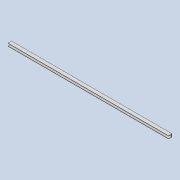
# Autodesk Inventor part: Decupare Heated Bed
Saved by Autodesk Inventor 2020 (Build 240168000, 168)
## iProperties
Created: 2021-01-16
Part Number: Decupare Heated Bed
Material: Generic
Document SubType Name: Modeling
Designer: Iulian Bors
Density: 1 g/cm^3
Appearance: Default
Author: Iulian Bors
Autodesk Inventor part; units mm, degrees
ref_plane "YZ Plane" through (0, 0, 0) normal (1, 0, 0) x (0, 1, 0)
ref_plane "XZ Plane" through (0, 0, 0) normal (0, 1, 0) x (-1, 0, 0)
ref_plane "XY Plane" through (0, 0, 0) normal (0, 0, 1) x (1, 0, 0)
sketch "Sketch1" plane through (0, 0, 0) normal (0, 0, 1) x (1, 0, 0)
  line L0 (-115, 2) -> (115, 2)
  line L1 (115, 2) -> (115, -2)
  line L2 (115, -2) -> (-115, -2)
  line L3 (-115, -2) -> (-115, 2)
  point P0 (0, 0)
  point P1 (-115, 0)
  point P2 (0, 2)
  dimension "d0" = 230
  dimension "d1" = 4
  constraints: 8 end point, 2 midpoint, 2 parallel, 1 horizontal, 1 horizontal alignment, 1 perpendicular, 1 vertical alignment
  measures "d0" distance of L0.start L0.end
  measures "d1" distance of L2.end L0.start
extrude "Extrusion1" add sketch "Sketch1" along normal blind 5
sketch "Sketch2" plane through (0, 0, 5) normal (0, 0, 1) x (1, 0, 0)
  line L0 (-118.277, 1.6) -> (118.277, 1.6)
  line L1 (118.277, 1.6) -> (118.277, -1.6)
  line L2 (118.277, -1.6) -> (-118.277, -1.6)
  line L3 (-118.277, -1.6) -> (-118.277, 1.6)
  point P0 (0, 0)
  point P1 (0, 1.6)
  point P2 (-118.277, 0)
  dimension "d4" = 3.2
  constraints: 8 end point, 2 midpoint, 2 parallel, 1 horizontal, 1 horizontal alignment, 1 perpendicular, 1 vertical alignment
  measures "d4" distance of L2.end L0.start
extrude "Extrusion2" cut sketch "Sketch2" against normal blind 4.5
body "Solid1"
